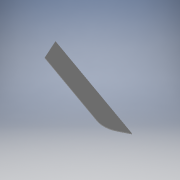
# Autodesk Inventor part: elevon
Saved by Autodesk Inventor 2017 (Build 210142000, 142)
## iProperties
Created: 2017-12-26
Part Number: elevon
Material: Generic
Document SubType Name: Modeling
Designer: will
Density: 1 g/cm^3
Appearance: Default
Author: will
Autodesk Inventor part; units mm, degrees
ref_plane "YZ Plane" through (0, 0, 0) normal (1, 0, 0) x (0, 1, 0)
ref_plane "XZ Plane" through (0, 0, 0) normal (0, 1, 0) x (-1, 0, 0)
ref_plane "XY Plane" through (0, 0, 0) normal (0, 0, 1) x (1, 0, 0)
sketch "Sketch1" plane through (0, 0, 0) normal (0, 0, 1) x (1, 0, 0)
  line L0 (299.9863, -338.0878) -> (344.1034, -353.6325)
  line L1 (299.9863, -338.0878) -> (299.9849, -338.2589)
  line L2 (343.7857, -353.6871) -> (299.9849, -338.2589)
  line L3 (344.1021, -353.7985) -> (343.7857, -353.6871)
  line L4 (387.9137, -369.2305) -> (344.1021, -353.7985)
  line L5 (388.2192, -369.3382) -> (387.9137, -369.2305)
  line L6 (432.0421, -384.7742) -> (388.2192, -369.3382)
  line L7 (432.3363, -384.8778) -> (432.0421, -384.7742)
  line L8 (476.1715, -400.3181) -> (432.3363, -384.8778)
  line L9 (476.4534, -400.4174) -> (476.1715, -400.3181)
  line L10 (520.3017, -415.8623) -> (476.4534, -400.4174)
  line L11 (520.5706, -415.9571) -> (520.3017, -415.8623)
  line L12 (564.4327, -431.4069) -> (520.5706, -415.9571)
  line L13 (564.6877, -431.4967) -> (564.4327, -431.4069)
  line L14 (608.5648, -446.9518) -> (564.6877, -431.4967)
  line L15 (608.8049, -447.0364) -> (608.5648, -446.9518)
  line L16 (652.6979, -462.4971) -> (608.8049, -447.0364)
  line L17 (652.922, -462.576) -> (652.6979, -462.4971)
  line L18 (696.8323, -478.0428) -> (652.922, -462.576)
  line L19 (697.0391, -478.1156) -> (696.8323, -478.0428)
  line L20 (740.9681, -493.589) -> (697.0391, -478.1156)
  line L21 (741.1562, -493.6553) -> (740.9681, -493.589)
  line L22 (785.1054, -509.1357) -> (741.1562, -493.6553)
  line L23 (785.2734, -509.1949) -> (785.1054, -509.1357)
  line L24 (829.2443, -524.6831) -> (785.2734, -509.1949)
  line L25 (829.3905, -524.7345) -> (829.2443, -524.6831)
  line L26 (873.3854, -540.2311) -> (829.3905, -524.7345)
  line L27 (873.5076, -540.2742) -> (873.3854, -540.2311)
  line L28 (917.5288, -555.78) -> (873.5076, -540.2742)
  line L29 (917.6248, -555.8138) -> (917.5288, -555.78)
  line L30 (961.6748, -571.3298) -> (917.6248, -555.8138)
  line L31 (961.742, -571.3535) -> (961.6748, -571.3298)
  line L32 (1005.8239, -586.8807) -> (961.742, -571.3535)
  line L33 (1005.859, -586.8931) -> (1005.8239, -586.8807)
  line L34 (1049.9762, -602.4327) -> (1005.859, -586.8931)
  line L35 (1049.9769, -602.3467) -> (1049.9762, -602.4327)
  line L36 (1006.0584, -586.8721) -> (1049.9769, -602.3467)
  line L37 (1005.8598, -586.8021) -> (1006.0584, -586.8721)
  line L38 (961.9186, -571.3194) -> (1005.8598, -586.8021)
  line L39 (961.7427, -571.2575) -> (961.9186, -571.3194)
  line L40 (917.7811, -555.7676) -> (961.7427, -571.2575)
  line L41 (917.6256, -555.7128) -> (917.7811, -555.7676)
  line L42 (873.6457, -540.2165) -> (917.6256, -555.7128)
  line L43 (873.5085, -540.1682) -> (873.6457, -540.2165)
  line L44 (829.512, -524.666) -> (873.5085, -540.1682)
  line L45 (829.3914, -524.6235) -> (829.512, -524.666)
  line L46 (785.3798, -509.116) -> (829.3914, -524.6235)
  line L47 (785.2743, -509.0789) -> (785.3798, -509.116)
  line L48 (741.249, -493.5666) -> (785.2743, -509.0789)
  line L49 (741.1572, -493.5342) -> (741.249, -493.5666)
  line L50 (697.1193, -478.0175) -> (741.1572, -493.5342)
  line L51 (697.0401, -477.9896) -> (697.1193, -478.0175)
  line L52 (652.9906, -462.4688) -> (697.0401, -477.9896)
  line L53 (652.923, -462.445) -> (652.9906, -462.4688)
  line L54 (608.8627, -446.9203) -> (652.923, -462.445)
  line L55 (608.806, -446.9003) -> (608.8627, -446.9203)
  line L56 (564.7358, -431.3722) -> (608.806, -446.9003)
  line L57 (564.6889, -431.3557) -> (564.7358, -431.3722)
  line L58 (520.6095, -415.8243) -> (564.6889, -431.3557)
  line L59 (520.5718, -415.811) -> (520.6095, -415.8243)
  line L60 (476.4838, -400.2767) -> (520.5718, -415.811)
  line L61 (476.4547, -400.2664) -> (476.4838, -400.2767)
  line L62 (432.3586, -384.7292) -> (476.4547, -400.2664)
  line L63 (432.3376, -384.7218) -> (432.3586, -384.7292)
  line L64 (388.2341, -369.1819) -> (432.3376, -384.7218)
  line L65 (388.2205, -369.1771) -> (388.2341, -369.1819)
  line L66 (344.11, -353.6348) -> (388.2205, -369.1771)
  line L67 (344.1034, -353.6325) -> (344.11, -353.6348)
  line L68 (299.9849, -338.2589) -> (354.5625, -460.6619)
  line L69 (354.5625, -460.6619) -> (929.3225, -663.1783)
  line L70 (929.3225, -663.1783) -> (1049.9769, -602.3467)
  constraints: 142 end point
extrude "Extrusion1" add sketch "Sketch1" along normal blind 5 contours L0 L67 L66 L65 L64 L63 L62 L61 L60 L59 L58 L57 L56 L55 L54 L53 L52 L51 L50 L49 L48 L47 L46 L45 L44 L43 L42 L41 L40 L39 L38 L37 L36 L70 L34 L33 L32 L31 L30 L29 L28 L27 L26 L25 L24 L23 L22 L21 L20 L19 L18 L17 L16 L15 L14 L13 L12 L11 L10 L9 L8 L7 L6 L5 L4 L3 L2 L1 | L2 L3 L4 L5 L6 L7 L8 L9 L10 L11 L12 L13 L14 L15 L16 L17 L18 L19 L20 L21 L22 L23 L24 L25 L26 L27 L28 L29 L30 L31 L32 L33 L34 L70 L69 L68
fillet "Fillet1" radius 153.25 1 edges at (929.3225, -663.1783, 2.5)
body "Solid1"
